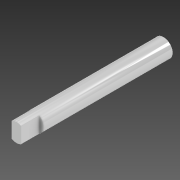
# Autodesk Inventor part: as bevelgear
Saved by Autodesk Inventor 2020 (Build 240168000, 168)
## iProperties
Created: 2020-05-19
Part Number: as bevelgear
Material: Generic
Document SubType Name: Modeling
Designer: stefa
Density: 1 g/cm^3
Appearance: Aluminum - Polished
Author: stefa
Autodesk Inventor part; units mm, degrees
ref_plane "YZ Plane" through (0, 0, 0) normal (1, 0, 0) x (0, 1, 0)
ref_plane "XZ Plane" through (0, 0, 0) normal (0, 1, 0) x (-1, 0, 0)
ref_plane "XY Plane" through (0, 0, 0) normal (0, 0, 1) x (1, 0, 0)
sketch "Sketch1" plane through (0, 0, 0) normal (0, 0, 1) x (1, 0, 0)
  circle A0 centre (0, 0) radius 4
  dimension "d0" = 8
  constraints: 1 centre point, 1 coincident
  measures "d0" diameter of A0
extrude "Extrusion1" add sketch "Sketch1" along normal blind 65
sketch "Sketch2" plane through (0, 0, 65) normal (0, 0, 1) x (1, 0, 0)
  circle A0 centre (0, 0) radius 4 projected
  line L0 (-2, -3.4641) -> (2, -3.4641)
  line L1 (2, -3.4641) -> (2, 3.4641)
  line L2 (2, 3.4641) -> (-2, 3.4641)
  line L3 (-2, 3.4641) -> (-2, -3.4641)
  line L4 (-2, -3.4641) -> (2, 3.4641) construction
  line L5 (2, -3.4641) -> (-2, 3.4641) construction
  circle A1 centre (0, 0) radius 4
  dimension "d3" = 4
  constraints: 12 end point, 2 midpoint, 2 parallel, 1 centre point, 1 coincident, 1 concentric, 1 horizontal, 1 perpendicular, 1 point on circle
  measures "d3" distance of L1.end L2.end
extrude "Extrusion2" cut sketch "Sketch2" against normal blind 8 contours A0 L1 | L3 A0
body "Solid1"
